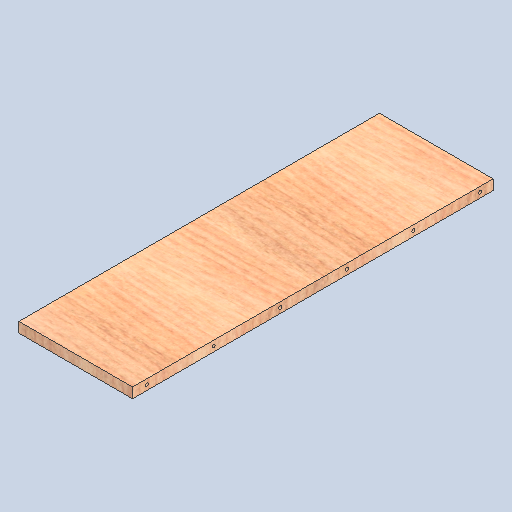
# Autodesk Inventor part: belt support
Saved by Autodesk Inventor 2023 (Build 270158000, 158)
## iProperties
Created: 2022-06-05
Part Number: belt support
Material: Wood (Birch)
Document SubType Name: Modeling
Designer: prana_p9lsmih
Density: 0.55 g/cm^3
Appearance: Birch - Natural Polished
Author: prana_p9lsmih
Autodesk Inventor part; units mm, degrees
ref_plane "YZ Plane" through (0, 0, 0) normal (1, 0, 0) x (0, 1, 0)
ref_plane "XZ Plane" through (0, 0, 0) normal (0, 1, 0) x (-1, 0, 0)
ref_plane "XY Plane" through (0, 0, 0) normal (0, 0, 1) x (1, 0, 0)
sketch "Sketch1" plane through (0, 0, 0) normal (0, 1, 0) x (-1, 0, 0)
  line L0 (0, 0) -> (145, 0)
  line L1 (145, 0) -> (145, -460)
  line L2 (145, -460) -> (0, -460)
  line L3 (0, -460) -> (0, 0)
  dimension "d0" = 145
  dimension "d1" = 460
  constraints: 8 end point, 2 parallel, 1 horizontal, 1 perpendicular
  measures "d0" distance of L1.end L2.end
  measures "d1" distance of L0.end L1.end
extrude "Extrusion1" add sketch "Sketch1" along normal blind 13
sketch "Sketch2" plane through (0, 0, 0) normal (1, 0, 0) x (0, 0, -1)
  line L0 (0, 0) -> (0, 13) projected
  line L1 (0, 13) -> (460, 13) projected
  point P0 (18.372, 6.5)
  dimension "d4" = 18.372
  dimension "d5" = 6.5
  measures "d4" distance from line of L0 point (18.372, 6.5)
  measures "d5" distance from line of L1 point (18.372, 6.5)
hole "Hole1" at (0, 6.5, -18.372) direction (-1, 0, 0) diameter 4 end through all
pattern_linear "Rectangular Pattern1" count 6 spacing 85 along (0, 0, -1) of "Hole1"
body "Solid1"
